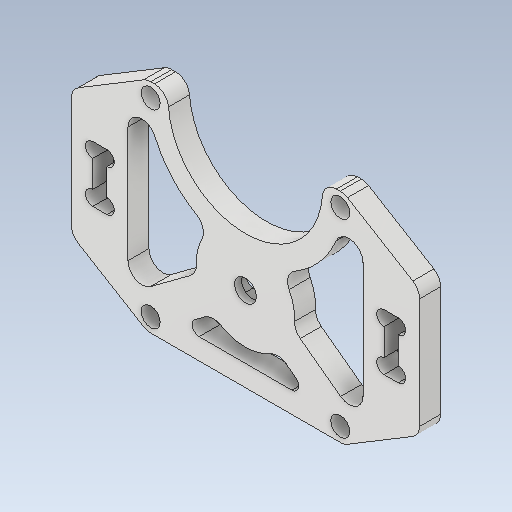
# Autodesk Inventor part: 付け根_メインフレーム_6_1
Saved by Autodesk Inventor 2020 (Build 240168000, 168)
## iProperties
Created: 2016-08-24
Part Number: 付け根_メインフレーム_6_1
Material: アルミニウム 2014-T4
Document SubType Name: Modeling
Designer: hiro
Density: 2.8 g/cm^3
Appearance: サテン
Mass: 6.34029 g
Surface Area: 27.1126 cm^2
Volume: 2.26439 cm^3
Category: 付け根
Author: hiro
Autodesk Inventor part; units mm, degrees
ref_plane "YZ Plane" through (0, 0, 0) normal (1, 0, 0) x (0, 1, 0)
ref_plane "XZ Plane" through (0, 0, 0) normal (0, 1, 0) x (-1, 0, 0)
ref_plane "XY Plane" through (0, 0, 0) normal (0, 0, 1) x (1, 0, 0)
derived "付け根_基準フレーム_6_1.ipt"
sketch "スケッチ1" plane through (0, 0, 0) normal (0, 0, 1) x (1, 0, 0)
  circle A0 centre (0, 0) radius 11 construction
  circle A1 centre (-13.5, -1) radius 1.35
  line L0 (-13.5, -1) -> (13.5, -1) construction
  line L1 (13.5, -1) -> (13.5, -28) construction
  line L2 (13.5, -28) -> (-13.5, -28) construction
  line L3 (-13.5, -28) -> (-13.5, -1) construction
  circle A2 centre (13.5, -1) radius 1.35
  circle A3 centre (-13.5, -28) radius 1.35
  circle A4 centre (13.5, -28) radius 1.35
  line L4 (0, 18) -> (0, -18) construction
  circle A5 centre (0, -18) radius 7 construction
  line L5 (-12.5, 29.5) -> (-12.5, 24.5) construction
  line L6 (-12.5, 24.5) -> (-7.9564, -18.8342) construction
  line L7 (-12.5, 29.5) -> (12.5, 29.5) construction
  line L8 (12.5, 29.5) -> (12.5, 24.5) construction
  line L9 (12.5, 24.5) -> (7.9564, -18.8342) construction
  arc A6 (-7.9564, -18.8342) -> (7.9564, -18.8342) centre (0, -18) ccw construction
  circle A7 centre (-9.5, 27) radius 1.55 construction
  circle A8 centre (9.5, 27) radius 1.55 construction
  line L10 (-5.51, 27.01) -> (5.51, 27.01) construction
  line L11 (5.51, 27.01) -> (5.51, 24.49) construction
  line L12 (5.51, 24.49) -> (-5.51, 24.49) construction
  line L13 (-5.51, 24.49) -> (-5.51, 27.01) construction
  circle A9 centre (-4.46, 27.01) radius 1.05 construction
  circle A10 centre (-4.46, 24.49) radius 1.05 construction
  circle A11 centre (4.46, 27.01) radius 1.05 construction
  circle A12 centre (4.46, 24.49) radius 1.05 construction
  line L14 (5.5, 27) -> (-5.5, 27) construction
  line L15 (-5.5, 27) -> (-5.5, 24.5) construction
  line L16 (-5.5, 24.5) -> (5.5, 24.5) construction
  line L17 (5.5, 24.5) -> (5.5, 27) construction
  circle A13 centre (0, -18) radius 5.55 construction
  circle A14 centre (0, 8.5) radius 1.35 construction
  circle A15 centre (-8.5, 0) radius 1.35 construction
  circle A16 centre (0, -8.5) radius 1.35 construction
  circle A17 centre (8.5, 0) radius 1.35 construction
  circle A18 centre (0, 0) radius 5.05 construction
  line L18 (-9.9856, 4.6139) -> (-3.1318, 19.4471) construction
  line L19 (3.1318, 19.4471) -> (9.9856, 4.6139) construction
  arc A19 (-9.9856, 4.6139) -> (9.9856, 4.6139) centre (0, 0) ccw construction
  arc A20 (3.1318, 19.4471) -> (-3.1318, 19.4471) centre (0, 18) ccw construction
  circle A21 centre (0, 18) radius 1.55 construction
  line L20 (-10.9545, 1) -> (-14.0575, 1)
  line L21 (-14.0575, 1) -> (-24.81, -5.5)
  line L22 (-24.81, -5.5) -> (-24.81, -23.5)
  line L23 (-24.81, -23.5) -> (-14.0575, -30)
  line L24 (-14.0575, -30) -> (14.0575, -30)
  line L25 (14.0575, -30) -> (24.81, -23.5)
  line L26 (24.81, -23.5) -> (24.81, -5.5)
  line L27 (24.81, -5.5) -> (14.0575, 1)
  line L28 (14.0575, 1) -> (10.9545, 1)
  arc A22 (-10.9545, 1) -> (10.9545, 1) centre (0, 0) ccw
  line L29 (-21.76, -10.49) -> (-19.74, -10.49)
  line L30 (-19.74, -10.49) -> (-19.74, -18.51)
  line L31 (-19.74, -18.51) -> (-21.76, -18.51)
  line L32 (-21.76, -18.51) -> (-21.76, -10.49)
  line L33 (-19.75, -10.5) -> (-21.75, -10.5) construction
  line L34 (-21.75, -10.5) -> (-21.75, -18.5) construction
  line L35 (-21.75, -18.5) -> (-19.75, -18.5) construction
  line L36 (-19.75, -18.5) -> (-19.75, -10.5) construction
  circle A23 centre (-21.76, -11.54) radius 1.05
  circle A24 centre (-19.74, -11.54) radius 1.05
  circle A25 centre (-19.74, -17.46) radius 1.05
  circle A26 centre (-21.76, -17.46) radius 1.05
  circle A27 centre (-13.5, -1) radius 2 construction
  line L37 (-24.81, -14.5) -> (-19.75, -14.5) construction
  circle A28 centre (-21.76, -11.54) radius 3.05 construction
  circle A29 centre (-13.5, -28) radius 2 construction
  line L38 (21.76, -10.49) -> (19.74, -10.49)
  line L39 (19.75, -10.5) -> (21.75, -10.5) construction
  circle A30 centre (19.74, -11.54) radius 1.05
  circle A31 centre (21.76, -11.54) radius 1.05
  circle A32 centre (21.76, -11.54) radius 3.05 construction
  line L40 (24.81, -14.5) -> (19.75, -14.5) construction
  line L41 (19.75, -18.5) -> (19.75, -10.5) construction
  line L42 (21.75, -10.5) -> (21.75, -18.5) construction
  line L43 (19.74, -10.49) -> (19.74, -18.51)
  line L44 (21.76, -18.51) -> (21.76, -10.49)
  circle A33 centre (19.74, -17.46) radius 1.05
  line L45 (21.75, -18.5) -> (19.75, -18.5) construction
  line L46 (19.74, -18.51) -> (21.76, -18.51)
  circle A34 centre (21.76, -17.46) radius 1.05
  line L47 (0, -14.7668) -> (2.8, -16.3834) construction
  line L48 (2.8, -16.3834) -> (2.8, -19.6166) construction
  line L49 (2.8, -19.6166) -> (0, -21.2332) construction
  line L50 (0, -21.2332) -> (-2.8, -19.6166) construction
  line L51 (-2.8, -19.6166) -> (-2.8, -16.3834) construction
  line L52 (-2.8, -16.3834) -> (0, -14.7668) construction
  line L53 (-19.75, 12) -> (19.75, 12) construction
  line L54 (19.75, 12) -> (19.75, -39.5) construction
  line L55 (19.75, -39.5) -> (-19.75, -39.5) construction
  line L56 (-19.75, -39.5) -> (-19.75, 12) construction
  arc A35 (3.5, 18) -> (-3.5, 18) centre (0, 18) ccw construction
  line L57 (-3.5, 18) -> (-3.5, 7.4558) construction
  line L58 (3.5, 18) -> (3.5, 7.4558) construction
  arc A36 (-3.5, 7.4558) -> (3.5, 7.4558) centre (0, 7.4558) ccw construction
  circle A37 centre (0, 18) radius 6.5 construction
  circle A38 centre (0, -18) radius 1.55
  line L59 (-21.75, -2) -> (-19.75, -2) construction
  line L60 (-19.75, -2) -> (-19.75, -27) construction
  line L61 (-19.75, -27) -> (-21.75, -27) construction
  line L62 (-21.75, -27) -> (-21.75, -2) construction
  circle A39 centre (0, -18) radius 36 construction
  line L63 (0, -18) -> (-25.4558, 7.4558) construction
  circle A40 centre (0, 0) radius 18 construction
  line L64 (-18, 0) -> (-25.4558, 7.4558) construction
  point P0 (0, -1)
  point P1 (0, 29.5)
  point P2 (-12.5, 27)
  point P3 (-21.75, -14.5)
  dimension "d1" = 3.1
  measures "d1" diameter of A38
extrude "押し出し1" add sketch "スケッチ1" along normal blind 3
sketch "スケッチ3" plane through (0, 0, 0) normal (0, 0, -1) x (-1, 0, 0)
  circle A0 centre (0, -18) radius 1.55 projected
  line L0 (-2.8, -16.3834) -> (0, -14.7668)
  line L1 (0, -14.7668) -> (2.8, -16.3834)
  line L2 (2.8, -16.3834) -> (2.8, -19.6166)
  line L3 (2.8, -19.6166) -> (0, -21.2332)
  line L4 (0, -21.2332) -> (-2.8, -19.6166)
  line L5 (-2.8, -19.6166) -> (-2.8, -16.3834)
  circle A1 centre (0, -20.1832) radius 1.05
  circle A2 centre (1.8907, -19.0916) radius 1.05
  circle A3 centre (1.8907, -16.9084) radius 1.05
  circle A4 centre (0, -15.8168) radius 1.05
  circle A5 centre (-1.8907, -16.9084) radius 1.05
  circle A6 centre (-1.8907, -19.0916) radius 1.05
  point P0 (2.8, -16.3834)
  point P1 (0, -14.7668)
  point P2 (-2.8, -16.3834)
  point P3 (-2.8, -19.6166)
  dimension "d5" = 2.1
  dimension "d4" = 5.6
  dimension "d8" = 360
  constraints: 12 end point, 3 vertical alignment, 1 coincident, 1 vertical, 48 other
  measures "d4" distance between parallel lines of L2 L5
extrude "押し出し2" cut sketch "スケッチ3" against normal blind 2 contours A0 A3 L2 A2 | A3 A0 | A0 A3 L1 L2 | A2 L2 L3 A0 | A0 A2 | A0 A4 L1 A3 | L2 A3 | A2 L3 A1 A0 | A2 L2 | A4 A0 | A0 A4 L0 L1 | A3 L1 | A1 L3 L4 A0 | A0 A1 | L3 A2 | A0 A5 L0 A4 | L1 A4 | A1 L4 A6 A0 | A1 L3 | A5 A0 | A0 A5 L5 L0 | A4 L0 | A6 L4 L5 A0 | A0 A6 | L4 A1 | A0 A6 L5 A5 | L0 A5 | A6 L4 | A5 L5 | L5 A6
sketch "スケッチ4" plane through (0, 0, 3) normal (0, 0, 1) x (1, 0, 0)
  line L0 (-19.74, -18.51) -> (-21.76, -18.51) projected
  arc A0 (-21.76, -16.41) -> (-21.76, -18.51) centre (-21.76, -17.46) ccw projected
  line L1 (-21.76, -16.41) -> (-21.76, -12.59) projected
  arc A1 (-21.76, -10.49) -> (-21.76, -12.59) centre (-21.76, -11.54) ccw projected
  line L2 (-21.76, -10.49) -> (-19.74, -10.49) projected
  arc A2 (-19.74, -12.59) -> (-19.74, -10.49) centre (-19.74, -11.54) ccw projected
  line L3 (-19.74, -12.59) -> (-19.74, -16.41) projected
  arc A3 (-19.74, -18.51) -> (-19.74, -16.41) centre (-19.74, -17.46) ccw projected
  circle A4 centre (0, -18) radius 1.55 projected
  circle A5 centre (13.5, -28) radius 1.35 projected
  circle A6 centre (-13.5, -28) radius 1.35 projected
  circle A7 centre (-13.5, -1) radius 1.35 projected
  line L4 (-14.0575, -30) -> (14.0575, -30) projected
  arc A8 (-10.9545, 1) -> (10.9545, 1) centre (0, 0) ccw projected
  line L5 (-9.63, -27) -> (9.63, -27)
  line L6 (9.63, -27) -> (4.6014, -23.2751)
  line L7 (-9.63, -27) -> (-4.6014, -23.2751)
  arc A9 (-2.9399, -22.0444) -> (2.9399, -22.0444) centre (0, -18) ccw construction
  line L8 (0, -18) -> (-13.5, -28) construction
  line L9 (0, -18) -> (13.5, -28) construction
  line L10 (-16.745, -4) -> (-16.745, -26.6703)
  line L11 (-16.745, -26.6703) -> (-6.8678, -19.3539)
  line L12 (-16.745, -4) -> (-13.4164, -4)
  arc A10 (-13.4164, -4) -> (-4.9826, -13.0833) centre (0, 0) ccw
  line L13 (-19.74, -10.495) -> (-21.76, -10.495) construction
  arc A11 (-21.76, -10.495) -> (-21.755, -12.585) centre (-21.76, -11.54) ccw construction
  line L14 (-21.755, -12.585) -> (-21.755, -16.415) construction
  arc A12 (-21.755, -16.415) -> (-21.76, -18.505) centre (-21.76, -17.46) ccw construction
  line L15 (-21.76, -18.505) -> (-19.74, -18.505) construction
  arc A13 (-19.74, -18.505) -> (-19.745, -16.415) centre (-19.74, -17.46) ccw construction
  line L16 (-19.745, -16.415) -> (-19.745, -12.585) construction
  arc A14 (-19.745, -12.585) -> (-19.74, -10.495) centre (-19.74, -11.54) ccw construction
  line L17 (0, 0) -> (0, -18) construction
  line L18 (16.745, -4) -> (16.745, -26.6703)
  line L19 (16.745, -26.6703) -> (6.8678, -19.3539)
  line L20 (16.745, -4) -> (13.4164, -4)
  arc A15 (3, -13.6748) -> (4.9826, -13.0833) centre (0, 0) ccw construction
  line L21 (-3, -13.6748) -> (-3, -16.4888) construction
  line L22 (3, -13.6748) -> (3, -16.4888) construction
  circle A16 centre (0, -18) radius 7 construction
  arc A17 (6.8678, -19.3539) -> (4.9826, -13.0833) centre (0, -18) ccw
  arc A18 (-4.6014, -23.2751) -> (4.6014, -23.2751) centre (0, -18) ccw
  arc A19 (-4.9826, -13.0833) -> (-6.8678, -19.3539) centre (0, -18) ccw
  arc A20 (-4.9826, -13.0833) -> (-3, -13.6748) centre (0, 0) ccw construction
  line L23 (-6.8678, -19.3539) -> (-3, -16.4888) construction
  line L24 (-4.6014, -23.2751) -> (-2.9399, -22.0444) construction
  line L25 (4.6014, -23.2751) -> (2.9399, -22.0444) construction
  line L26 (6.8678, -19.3539) -> (3, -16.4888) construction
  arc A21 (4.9826, -13.0833) -> (13.4164, -4) centre (0, 0) ccw
  dimension "d13" = 5
  dimension "d14" = 3
  dimension "d15" = 1.5
  dimension "d16" = 3
  dimension "d17" = 3
  dimension "d18" = 0.005
  dimension "d19" = 3
  dimension "d20" = 3
  dimension "d24" = 3
  dimension "d25" = 1.5
  constraints: 44 end point, 30 point on circle, 13 centre point, 7 parallel, 6 coincident, 4 symmetric about line, 3 vertical, 2 horizontal, 1 collinear, 1 tangent, 8 other
  measures "d13" radius of A9
  measures "d14" distance between parallel lines of L5 L4
  measures "d15" distance between parallel lines of L8 L7
  measures "d16" radial gap between concentric circles of A8 A10
  measures "d17" distance between parallel lines of L8 L11
  measures "d18" distance between parallel lines of L2 L13
  measures "d19" distance between parallel lines of L10 L16
  measures "d20" distance from line of A7.centre L12
  measures "d24" distance between parallel lines of L17 L21
  measures "d25" distance between parallel lines of L6 L9
extrude "押し出し3" cut sketch "スケッチ4" against normal blind 3 contours L7 A18 L6 L5 | L12 A10 A19 L11 L10 | L18 L19 A17 A21 L20
fillet "フィレット2" radius 2 22 edges at (-16.745, -4, 1.5) (-13.4164, -4, 1.5) (-10.9545, 1, 1.5) (-14.0575, 1, 1.5) (-24.81, -5.5, 1.5) (-24.81, -23.5, 1.5) (-16.745, -26.6703, 1.5) (10.9545, 1, 1.5) (14.0575, 1, 1.5) (16.745, -4, 1.5) (13.4164, -4, 1.5) (24.81, -5.5, 1.5) (24.81, -23.5, 1.5) (16.745, -26.6703, 1.5) (14.0575, -30, 1.5) (-14.0575, -30, 1.5) (-4.9826, -13.0833, 1.5) (-6.8678, -19.3539, 1.5) (-4.6014, -23.2751, 1.5) (4.6014, -23.2751, 1.5) (4.9826, -13.0833, 1.5) (6.8678, -19.3539, 1.5)
fillet "フィレット2" radius 1 2 edges at (-9.63, -27, 1.5) (9.63, -27, 1.5)
equation "\"d25\" = d15"
